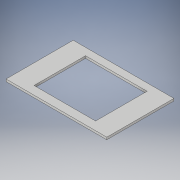
# Autodesk Inventor part: Table_plate
Saved by Autodesk Inventor 2019.4 (Build 234330000, 330)
## iProperties
Created: 2019-12-14
Part Number: Table_plate
Material: Generic
Document SubType Name: Modeling
Designer: fabfarm
Density: 1 g/cm^3
Appearance: Default
Author: fabfarm
Autodesk Inventor part; units mm, degrees
ref_plane "YZ Plane" through (0, 0, 0) normal (1, 0, 0) x (0, 1, 0)
ref_plane "XZ Plane" through (0, 0, 0) normal (0, 1, 0) x (-1, 0, 0)
ref_plane "XY Plane" through (0, 0, 0) normal (0, 0, 1) x (1, 0, 0)
sketch "Sketch1" plane through (0, 0, 0) normal (0, 1, 0) x (-1, 0, 0)
  line L0 (0, 0) -> (900, 0)
  line L1 (900, 0) -> (900, -600)
  line L2 (900, -600) -> (0, -600)
  line L3 (0, -600) -> (0, 0)
  line L4 (725, -75) -> (175, -75)
  line L5 (175, -75) -> (175, -535)
  line L6 (175, -535) -> (725, -535)
  line L7 (725, -535) -> (725, -75)
  dimension "d0" = 900
  dimension "d1" = 600
  dimension "d23" = 175
  dimension "d24" = 75
  dimension "d25" = 460
  dimension "d26" = 550
  constraints: 16 end point, 4 parallel, 2 horizontal, 2 perpendicular
  measures "d0" distance of L0.start L0.end
  measures "d1" distance between parallel lines of L0 L2
  measures "d23" distance between parallel lines of L3 L5
  measures "d24" distance between parallel lines of L0 L4
  measures "d25" distance of L4.end L5.end
  measures "d26" distance of L4.start L4.end
extrude "Extrusion4" add sketch "Sketch1" along normal blind 20.18
body "Solid2"
